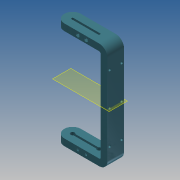
# Autodesk Inventor part: slide frame
Saved by Autodesk Inventor 2013 (Build 170138000, 138)
## iProperties
Created: 2017-03-30
Part Number: slide frame
Material: Generic
Document SubType Name: Modeling
Designer: employee
Density: 1 g/cm^3
Author: employee
Autodesk Inventor part; units mm, degrees
ref_plane "YZ Plane" through (0, 0, 0) normal (1, 0, 0) x (0, 1, 0)
ref_plane "XZ Plane" through (0, 0, 0) normal (0, 1, 0) x (-1, 0, 0)
ref_plane "XY Plane" through (0, 0, 0) normal (0, 0, 1) x (1, 0, 0)
sketch "Sketch1" plane through (0, 0, 0) normal (0, 0, 1) x (1, 0, 0)
  line L0 (0, 12.5) -> (65, 12.5)
  line L1 (65, 12.5) -> (65, -12.5)
  line L2 (65, -12.5) -> (0, -12.5)
  arc A0 (0, 12.5) -> (0, -12.5) centre (0, 0) ccw
  dimension "d0" = 65
  dimension "d2" = 25
  constraints: 6 end point, 2 point on circle, 2 tangent, 1 centre point, 1 coincident, 1 horizontal, 1 parallel, 1 perpendicular
  measures "d0" distance of L1.end L2.end
  measures "d2" distance between parallel lines of L0 L2
extrude "Extrusion1" add sketch "Sketch1" along normal blind 10
sketch "Sketch2" plane through (65, -12.5, 0) normal (1, 0, 0) x (0, 0, -1)
  line L0 (0, 25) -> (0, 0) projected
  line L1 (0, 25) -> (-10, 25) projected
  line L2 (0, 0) -> (-10, 0) projected
  line L3 (-10, 25) -> (150, 25)
  line L4 (150, 25) -> (150, 0)
  line L5 (150, 0) -> (-10, 0)
  line L6 (-10, 0) -> (-10, 25)
  point P0 (0, 12.5)
  dimension "d5" = 160
  constraints: 8 end point, 2 parallel, 1 horizontal, 1 perpendicular
  measures "d5" distance of L4.end L2.end
extrude "Extrusion2" add sketch "Sketch2" against normal blind 10 contours L3 L4 L5 L0
sketch "Sketch3" plane through (65, -12.5, -150) normal (0, 0, -1) x (-1, 0, 0)
  line L0 (10, 25) -> (10, 0) projected
  line L1 (10, 0) -> (65, 0) projected
  arc A0 (65, 0) -> (65, 25) centre (65, 12.5) ccw projected
  line L2 (65, 25) -> (10, 25) projected
extrude "Extrusion3" add sketch "Sketch3" against normal blind 10
sketch "Sketch4" plane through (0, 0, 0) normal (0, 0, -1) x (-1, 0, 0)
  arc A0 (0, -12.5) -> (0, 12.5) centre (0, 0) ccw projected
  circle A1 centre (0, 0) radius 3
  circle A2 centre (-40, 0) radius 3
  dimension "d10" = 6
  dimension "d14" = 40
  constraints: 2 centre point, 1 coincident, 1 equal radius, 1 horizontal alignment
  measures "d10" diameter of A1
  measures "d14" distance of A0.centre A2.centre
extrude "Extrusion4" cut sketch "Sketch4" against normal blind 5 and the other way blind 150
fillet "Fillet2" radius 2.5 2 edges at (55, 0, -140) (55, 0, 0)
fillet "Fillet2" radius 12.5 2 edges at (65, 0, 10) (65, 0, -150)
sketch "Sketch11" plane through (55, -12.5, 0) normal (-1, 0, 0) x (0, 0, 1)
  line L0 (-140, 0) -> (-137.5, 0) projected
  line L1 (-137.5, 0) -> (-137.5, 25) projected
  line L2 (-137.5, 25) -> (-140, 25) projected
  line L3 (-140, 25) -> (-140, 0) projected
  line L4 (-120, 21.5) -> (-120, 3.5)
  line L5 (-140, 0) -> (-140, 25) projected
  circle A0 centre (-120, 21.5) radius 1.75
  circle A1 centre (-120, 3.5) radius 1.75
  point P0 (0, 12.5)
  point P1 (-140, 12.5)
  point P2 (-120, 12.5)
  dimension "d49" = 20
  dimension "d50" = 3.5
  dimension "d51" = 18
  constraints: 2 centre point, 2 coincident, 2 end point, 2 midpoint, 1 equal radius, 1 horizontal alignment, 1 parallel
  measures "d49" distance between parallel lines of L4 L3
  measures "d50" diameter of A0
  measures "d51" distance of L4.start L4.end
extrude "Extrusion11" cut sketch "Sketch11" against normal through all contours A0 | A1
sketch "Sketch12" plane through (55, -12.5, 0) normal (-1, 0, 0) x (0, 0, 1)
  circle A0 centre (-120, 21.5) radius 1.75 projected
  circle A1 centre (-120, 3.5) radius 1.75 projected
  line L0 (-123.1754, 21.5) -> (-121.5877, 24.25)
  line L1 (-121.5877, 24.25) -> (-118.4123, 24.25)
  line L2 (-118.4123, 24.25) -> (-116.8246, 21.5)
  line L3 (-116.8246, 21.5) -> (-118.4123, 18.75)
  line L4 (-118.4123, 18.75) -> (-121.5877, 18.75)
  line L5 (-121.5877, 18.75) -> (-123.1754, 21.5)
  line L6 (-123.1754, 3.5) -> (-121.5877, 6.25)
  line L7 (-121.5877, 6.25) -> (-118.4123, 6.25)
  line L8 (-118.4123, 6.25) -> (-116.8246, 3.5)
  line L9 (-116.8246, 3.5) -> (-118.4123, 0.75)
  line L10 (-118.4123, 0.75) -> (-121.5877, 0.75)
  line L11 (-121.5877, 0.75) -> (-123.1754, 3.5)
  point P0 (0, 12.5)
  dimension "d54" = 5.5
  constraints: 24 end point, 2 coincident, 2 horizontal, 1 parallel, 26 other
  measures "d54" distance between parallel lines of L1 L4
extrude "Extrusion12" cut sketch "Sketch12" against normal blind 4
sketch "Sketch13" plane through (0, 0, -150) normal (0, 0, -1) x (-1, 0, 0)
  line L0 (-52.5, 12.5) -> (0, 12.5) projected
  circle A0 centre (0, 0) radius 3 projected
  circle A1 centre (-40, 0) radius 3 projected
  line L1 (-40, 1.5) -> (0, 1.5)
  arc A2 (0, -1.5) -> (0, 1.5) centre (0, 0) ccw
  line L2 (0, -1.5) -> (-40, -1.5)
  arc A3 (-40, 1.5) -> (-40, -1.5) centre (-40, 0) ccw
  dimension "d57" = 3
  constraints: 4 end point, 4 point on circle, 4 tangent, 2 centre point, 2 parallel, 1 coincident, 1 concentric
  measures "d57" distance between parallel lines of L1 L2
extrude "Extrusion13" cut sketch "Sketch13" against normal through all contours L1 A2 L2 A0 | A0 L2 A1 L1 | A1 L2 A3 L1 picked at (-0.9945, 0.1045) picked at (-39, 0)
sketch "Sketch14" plane through (0, 12.5, 10) normal (0, 1, 0) x (1, 0, 0)
  line L0 (0, 10) -> (0, 0) projected
  line L1 (65, 147.5) -> (65, 12.5) projected
  circle A0 centre (21.125, 5) radius 1.75
  circle A1 centre (33.625, 5) radius 1.75
  line L2 (21.125, 5) -> (33.625, 5)
  line L3 (43, 10) -> (43, 5) projected
  arc A2 (65, 147.5) -> (52.5, 160) centre (52.5, 147.5) ccw projected
  line L4 (52.5, 160) -> (0, 160) projected
  line L5 (0, 160) -> (0, 150) projected
  line L6 (52.5, 150) -> (0, 150) projected
  arc A3 (55, 147.5) -> (52.5, 150) centre (52.5, 147.5) ccw projected
  line L7 (55, 12.5) -> (55, 147.5) projected
  arc A4 (52.5, 10) -> (55, 12.5) centre (52.5, 12.5) ccw projected
  line L8 (0, 10) -> (52.5, 10) projected
  line L9 (52.5, 0) -> (0, 0) projected
  arc A5 (52.5, 0) -> (65, 12.5) centre (52.5, 12.5) ccw projected
  point P0 (0, 5)
  point P1 (27.375, 5)
  dimension "d61" = 12.5
  dimension "d63" = 3.5
  dimension "d79" = 15.625
  constraints: 2 centre point, 2 end point, 2 horizontal alignment, 2 midpoint, 1 equal radius, 1 perpendicular
  measures "d61" distance of L2.start L2.end
  measures "d63" diameter of A0
  measures "d79" distance from line of point (27.375, 5) L3
extrude "Extrusion14" cut sketch "Sketch14" against normal through all contours A0 | A1
pattern_linear "Rectangular Pattern1" count 2 spacing 150 along (0, 0, -1) of "Extrusion14"
sketch "Sketch15" plane through (0, -12.5, 0) normal (0, -1, 0) x (1, 0, 0)
  circle A0 centre (21.125, 5) radius 1.75 projected
  circle A1 centre (33.625, 5) radius 1.75 projected
  line L0 (23.875, 6.5877) -> (23.875, 3.4123)
  line L1 (23.875, 3.4123) -> (21.125, 1.8246)
  line L2 (21.125, 1.8246) -> (18.375, 3.4123)
  line L3 (18.375, 3.4123) -> (18.375, 6.5877)
  line L4 (18.375, 6.5877) -> (21.125, 8.1754)
  line L5 (21.125, 8.1754) -> (23.875, 6.5877)
  line L6 (36.375, 6.5877) -> (36.375, 3.4123)
  line L7 (36.375, 3.4123) -> (33.625, 1.8246)
  line L8 (33.625, 1.8246) -> (30.875, 3.4123)
  line L9 (30.875, 3.4123) -> (30.875, 6.5877)
  line L10 (30.875, 6.5877) -> (33.625, 8.1754)
  line L11 (33.625, 8.1754) -> (36.375, 6.5877)
  dimension "d70" = 5.5
  constraints: 24 end point, 2 coincident, 2 vertical, 1 parallel, 26 other
  measures "d70" distance between parallel lines of L3 L0
extrude "Extrusion15" cut sketch "Sketch15" against normal blind 4
sketch "Sketch16" plane through (0, 12.5, 10) normal (0, 1, 0) x (1, 0, 0)
  circle A0 centre (33.625, 155) radius 1.75 projected
  circle A1 centre (21.125, 155) radius 1.75 projected
  line L0 (21.125, 151.8246) -> (18.375, 153.4123)
  line L1 (18.375, 153.4123) -> (18.375, 156.5877)
  line L2 (18.375, 156.5877) -> (21.125, 158.1754)
  line L3 (21.125, 158.1754) -> (23.875, 156.5877)
  line L4 (23.875, 156.5877) -> (23.875, 153.4123)
  line L5 (23.875, 153.4123) -> (21.125, 151.8246)
  line L6 (33.625, 151.8246) -> (30.875, 153.4123)
  line L7 (30.875, 153.4123) -> (30.875, 156.5877)
  line L8 (30.875, 156.5877) -> (33.625, 158.1754)
  line L9 (33.625, 158.1754) -> (36.375, 156.5877)
  line L10 (36.375, 156.5877) -> (36.375, 153.4123)
  line L11 (36.375, 153.4123) -> (33.625, 151.8246)
  dimension "d73" = 5.5
  constraints: 24 end point, 2 coincident, 2 vertical, 1 parallel, 26 other
  measures "d73" distance between parallel lines of L1 L4
extrude "Extrusion16" cut sketch "Sketch16" against normal blind 4
ref_plane "Work Plane1" through (65, -12.5, -70) normal (0, 0, 1) x (1, 0, 0)
pattern_linear "Rectangular Pattern2" count 3 spacing 50 along (0, 0, 1) of "Extrusion11", "Extrusion12"
body "Solid1"
